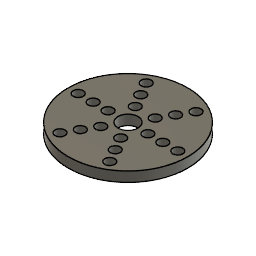
ex28aug29 (Autodesk Fusion 360 design; units mm, degrees)
part number: 2026-08-29-11-39-51-354
Autodesk Fusion 360 part; units mm, degrees
sketch "Sketch1" plane through (0, 0, 0) normal (0, 1, 0) x (1, 0, 0)
  circle A0 centre (0, 0) radius 60
  circle A1 centre (0, 0) radius 10
  circle A2 centre (0, 0) radius 20
  circle A3 centre (0, 0) radius 35
  circle A4 centre (0, 0) radius 50
  circle A5 centre (20, 0) radius 5
  circle A6 centre (35, 0) radius 5
  circle A7 centre (50, 0) radius 5
  circle A8 centre (10, 17.3205) radius 5
  circle A9 centre (17.5, 30.3109) radius 5
  circle A10 centre (25, 43.3013) radius 5
  circle A11 centre (-10, 17.3205) radius 5
  circle A12 centre (-17.5, 30.3109) radius 5
  circle A13 centre (-25, 43.3013) radius 5
  circle A14 centre (-20, 0) radius 5
  circle A15 centre (-35, 0) radius 5
  circle A16 centre (-50, 0) radius 5
  circle A17 centre (-10, -17.3205) radius 5
  circle A18 centre (-17.5, -30.3109) radius 5
  circle A19 centre (-25, -43.3013) radius 5
  circle A20 centre (10, -17.3205) radius 5
  circle A21 centre (17.5, -30.3109) radius 5
  circle A22 centre (25, -43.3013) radius 5
  dimension "d1" = 120
  dimension "d2" = 20
  dimension "d3" = 40
  dimension "d4" = 70
  dimension "d5" = 100
  dimension "d7" = 10
  dimension "d8" = 10
  dimension "d9" = 10
  dimension "d12" = 360
  constraint coincident A0.centre A1.centre
  constraint concentric A3 A4
  constraint coincident A2 A5.centre
  constraint coincident A3 A6.centre
  measures "d1" diameter of A0
  measures "d2" diameter of A1
  measures "d3" diameter of A2
  measures "d4" diameter of A3
  measures "d5" diameter of A4
  measures "d7" diameter of A5
  measures "d8" diameter of A6
  measures "d9" diameter of A7
extrude "Extrude1" add sketch "Sketch1" along normal blind 10 contours A0 | A2 A5 A8 A11 A14 A17 A20 | A3 A6 A9 A12 A15 A18 A21 | A4 A7 A10 A13 A16 A19 A22
